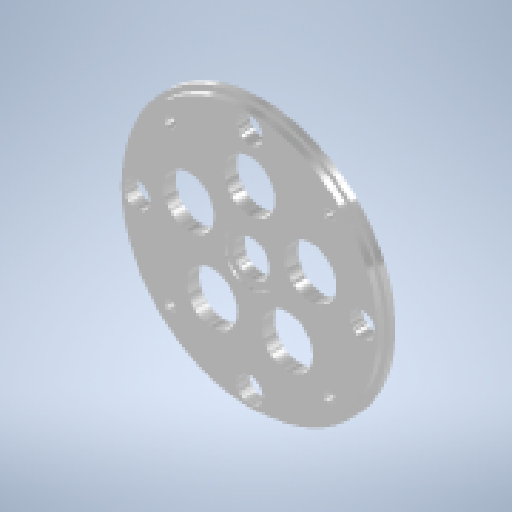
# Autodesk Inventor part: 出力板
Saved by Autodesk Inventor 2024 (Build 280153000, 153)
## iProperties
Created: 2023-05-29
Part Number: 出力板
Material: アルミニウム 6061
Document SubType Name: Modeling
Designer: yuta2
Density: 2.7 g/cm^3
Appearance: アルミニウム - フラット
Mass: 85.8137 g
Surface Area: 173.25 cm^2
Volume: 31.7829 cm^3
Author: yuta2
Autodesk Inventor part; units mm, degrees
ref_plane "YZ Plane" through (0, 0, 0) normal (1, 0, 0) x (0, 1, 0)
ref_plane "XZ Plane" through (0, 0, 0) normal (0, 1, 0) x (-1, 0, 0)
ref_plane "XY Plane" through (0, 0, 0) normal (0, 0, 1) x (1, 0, 0)
sketch "スケッチ1" plane through (0, 0, 0) normal (0, 0, 1) x (1, 0, 0)
  circle A0 centre (0, 0) radius 50
  dimension "d0" = 100
  constraints: 1 centre point, 1 coincident
  measures "d0" diameter of A0
extrude "押し出し1" add sketch "スケッチ1" along normal blind 2.5
sketch "スケッチ2" plane through (0, 0, 0) normal (0, 0, -1) x (-1, 0, 0)
  circle A0 centre (0, 0) radius 52
  dimension "d3" = 104
  constraints: 1 centre point, 1 coincident
  measures "d3" diameter of A0
extrude "押し出し2" add sketch "スケッチ2" along normal blind 2.5
sketch "スケッチ3" plane through (0, 0, -2.5) normal (0, 0, -1) x (-1, 0, 0)
  point P0 (0, 0)
  point P1 (0, 0)
  constraints: 1 coincident
hole "穴1" at (0, 0, -2.5) direction (0, 0, 1) diameter 14 end through all
sketch "スケッチ4" plane through (0, 0, 2.5) normal (0, 0, 1) x (1, 0, 0)
  point P0 (0, 0)
  point P1 (0, 44)
  dimension "d13" = 44
  constraints: 1 vertical alignment
  measures "d13" distance of point (0, 0) point (0, 44)
hole "穴2" at (0, 44, 2.5) direction (0, 0, -1) diameter 10 end through all
pattern_circular "円形状パターン1" count 4 over 360 about axis through (0, 0, 144.6632) along (0, 0, -1) of "穴2"
sketch "スケッチ5" plane through (0, 0, -2.5) normal (0, 0, -1) x (-1, 0, 0)
  circle A0 centre (28.7245, 26.8039) radius 17.2489
  circle A1 centre (0, -44) radius 5 projected
  circle A2 centre (0, 0) radius 44
  line L0 (31.1127, 31.1127) -> (0, 0)
  circle A3 centre (0, 44) radius 5 projected
  line L1 (0, 0) -> (0, 44)
  dimension "d24" = 45
  constraints: 4 end point, 2 centre point, 2 point on circle, 1 coincident, 1 vertical
  measures "d24" angle of L1 L0
hole "穴3" at (-31.1127, 31.1127, -2.5) direction (0, 0, 1) diameter 4.2 end through all
pattern_circular "円形状パターン2" count 4 over 360 about axis through (0, 0, 0) along (0, 0, -1) of "穴3"
sketch "スケッチ6" plane through (0, 0, 2.5) normal (0, 0, 1) x (1, 0, 0)
  circle A0 centre (0, 0) radius 35
  circle A1 centre (0, 0) radius 15
  circle A2 centre (0, 25) radius 10
  circle A3 centre (-23.7764, 7.7254) radius 10
  circle A4 centre (-14.6946, -20.2254) radius 10
  circle A5 centre (14.6946, -20.2254) radius 10
  circle A6 centre (23.7764, 7.7254) radius 10
  dimension "d35" = 70
  dimension "d36" = 30
  dimension "d39" = 360
  constraints: 7 centre point, 2 coincident, 2 tangent, 11 other
  measures "d35" diameter of A0
  measures "d36" diameter of A1
extrude "押し出し3" cut sketch "スケッチ6" against normal through all contours A6 | A5 | A2 | A4 | A3
sketch "スケッチ8" plane through (0, 0, 2.5) normal (0, 0, 1) x (1, 0, 0)
  circle A0 centre (0, 0) radius 10
  dimension "d46" = 20
  constraints: 1 centre point, 1 coincident
  measures "d46" diameter of A0
extrude "押し出し5" cut sketch "スケッチ8" against normal blind 0.8
